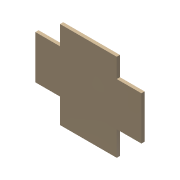
# Autodesk Inventor part: pcb_btm
Saved by Autodesk Inventor 2015 SP1 (Build 190203100, 203)
## iProperties
Created: 2015-12-08
Part Number: pcb_btm
Material: Полиэтилен, высокая плотность
Document SubType Name: Modeling
Designer: User
Density: 0.952 g/cm^3
Appearance: Гладкий — серовато-белый
Mass: 0.655105 g
Surface Area: 14.9671 cm^2
Volume: 0.688135 cm^3
Author: User
Autodesk Inventor part; units mm, degrees
ref_plane "YZ Plane" through (0, 0, 0) normal (1, 0, 0) x (0, 1, 0)
ref_plane "XZ Plane" through (0, 0, 0) normal (0, 1, 0) x (-1, 0, 0)
ref_plane "XY Plane" through (0, 0, 0) normal (0, 0, 1) x (1, 0, 0)
sketch "Эскиз1" plane through (0, 0, 0) normal (0, 1, 0) x (-1, 0, 0)
  line L0 (17.2838, -7.675) -> (-15.7162, -7.675)
  line L1 (-15.7162, -7.675) -> (-15.7162, 5.865)
  line L2 (-15.7162, 5.865) -> (17.2838, 5.865)
  line L3 (17.2838, 5.865) -> (17.2838, -7.675)
  line L4 (9.6038, -15.355) -> (-8.0362, -15.355)
  line L5 (-8.0362, -15.355) -> (-8.0362, 11.865)
  line L6 (-8.0362, 11.865) -> (9.6038, 11.865)
  line L7 (9.6038, 11.865) -> (9.6038, -15.355)
  point P0 (0, 0)
  dimension "d0" = 13.54
  dimension "d1" = 33
  dimension "d2" = 7.68
  dimension "d3" = 7.68
  dimension "d4" = 6
  dimension "d5" = 7.68
  constraints: 16 end point, 4 parallel, 2 horizontal, 2 perpendicular
  measures "d0" distance of L0.end L1.end
  measures "d1" distance of L1.end L2.end
  measures "d2" distance between parallel lines of L7 L3
  measures "d3" distance between parallel lines of L1 L5
  measures "d4" distance between parallel lines of L2 L6
  measures "d5" distance between parallel lines of L0 L4
extrude "Выдавливание1" add sketch "Эскиз1" along normal blind 1
equation "\"d3\" = d2"
equation "\"d5\" = d2"
